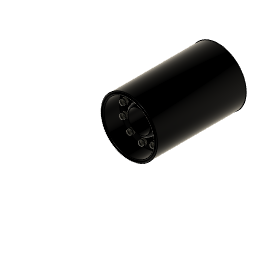
camera v2 (Autodesk Fusion 360 design; units mm, degrees)
Autodesk Fusion 360 part; units mm, degrees
cylinder "CylinderPrimitive1" add diameter 100 height 160 placed x (1, 0, 0) y (0, 0, -1) z (0, 1, 0) at (0, 0, 0) makes body 1
hole "Hole1" at (0, 0, 0) direction (0, 1, 0) diameter 90 depth 30 tip angle 180 bodies 1
cylinder "CylinderPrimitive2" add diameter 50 height 10 placed x (1, 0, 0) y (0, 0, 1) z (0, -1, 0) at (0, 30, 0) bodies 1
hole "Hole2" at (0, 20, 0) direction (0, 1, 0) diameter 40 depth 30 tip angle 180 bodies 1
cylinder "CylinderPrimitive3" add diameter 20 height 15 placed x (1, 0, 0) y (0, 0, 1) z (0, -1, 0) at (0, 50, 0) separate body makes body 2
fillet "Fillet1" radius 10 1 faces at (2.3712, 35, -3.5556) on bodies 2
cylinder "CylinderPrimitive4" add diameter 10 height 10 placed x (1, 0, 0) y (0, 0, 1) z (0, -1, 0) at (0, 30, 35) separate body makes body 3
fillet "Fillet2" radius 5 1 faces at (1.8073, 20, 36.9156) on bodies 3
pattern_circular "C-Pattern1" count 10 over 360 about axis through (0, -160, 0) along (0, 1, 0) of bodies 3 makes body 4 at (24.3048, 26.6667, 24.9885) makes body 5 at (34.3509, 28.3333, 5.9301) makes body 6 at (31.5068, 28.3333, -15.488) makes body 7 at (16.2549, 26.6667, -30.8372) makes body 8 at (-4.9752, 26.6667, -34.5022) makes body 9 at (-16.0438, 24.3474, -26.2993) makes body 10 at (-34.3509, 28.3333, -5.9301) makes body 11 at (-29.9699, 24.3474, 7.1317) makes body 12 at (-16.2549, 26.6667, 30.8372)
box "BoxPrimitive1" cut length 10 width 2 height -4 placed x (0, 0, 1) y (-1, 0, 0) z (0, -1, 0) at (-13, 50, -5) bodies 1
box "BoxPrimitive2" cut length 10 width 2 height -2 placed x (0, 0, 1) y (-1, 0, 0) z (0, -1, 0) at (15, 50, -5) bodies 1
copy_body "Body->Comp1" bodies 2 removing the originals makes body 13 in component "Component"
fillet "Fillet3" radius 7.5 1 edges at (-23.3082, 20, -9.0404) on bodies 1
fillet "Fillet4" radius 2.5 1 faces at (48.1052, 0, 3.605) on bodies 1
component "Component" placed x (1, 0, 0) y (0, 1, 0) z (0, 0, 1) at (0, 0, 0)
